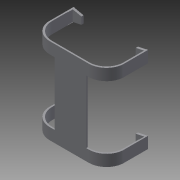
# Autodesk Inventor part: tapa
Saved by Autodesk Inventor 2013 (Build 170138000, 138)
## iProperties
Created: 2013-05-01
Part Number: tapa
Material: Generic
Document SubType Name: Modeling
Designer: otrab
Density: 1 g/cm^3
Author: otrab
Autodesk Inventor part; units mm, degrees
ref_plane "YZ Plane" through (0, 0, 0) normal (1, 0, 0) x (0, 1, 0)
ref_plane "XZ Plane" through (0, 0, 0) normal (0, 1, 0) x (-1, 0, 0)
ref_plane "XY Plane" through (0, 0, 0) normal (0, 0, 1) x (1, 0, 0)
sketch "Sketch1" plane through (0, 0, 0) normal (0, 1, 0) x (-1, 0, 0)
  line L0 (-26, -31) -> (26, -31)
  line L1 (26, -31) -> (26, 31)
  line L2 (26, 31) -> (-26, 31)
  line L3 (-26, 31) -> (-26, -31)
  line L4 (-26, -31) -> (26, 31) construction
  line L5 (26, -31) -> (-26, 31) construction
  point P0 (0, 0)
  dimension "d0" = 52
  dimension "d2" = 62
  constraints: 12 end point, 2 midpoint, 2 parallel, 1 horizontal, 1 perpendicular
  measures "d0" distance of L1.end L2.end
  measures "d2" distance of L2.end L0.start
extrude "Extrusion1" add sketch "Sketch1" along normal blind 1
sketch "Sketch2" plane through (0, 1, 0) normal (0, 1, 0) x (1, 0, 0)
  line L0 (26, 31) -> (-26, 31) projected
  line L1 (-26, 31) -> (-26, -31) projected
  line L2 (-26, -31) -> (26, -31) projected
  line L3 (-26, 31) -> (-25, 31)
  line L4 (-25, 31) -> (-25, -31)
  line L5 (-26, -31) -> (-25, -31)
  line L6 (-26, -31) -> (-26, 31)
  line L7 (0, 46.5401) -> (0, -49.8176) construction
  line L8 (26, 31) -> (26, -31)
  line L9 (26, 31) -> (25, 31)
  line L10 (25, 31) -> (25, -31)
  line L11 (26, -31) -> (25, -31)
  line L12 (26, -31) -> (26, 31)
  point P0 (0, 0)
  dimension "d5" = 1
  constraints: 20 end point, 3 perpendicular, 2 point on line, 2 symmetric about line, 1 parallel
  measures "d5" distance of L0.end L3.end
extrude "Extrusion2" add sketch "Sketch2" along normal blind 28 contours L8 L2 L10 L0 | L4 L2 L1 L0
fillet "Fillet1" radius 12 1 edges at (-25, 1, 0)
mirror "Mirror1" about plane through (0, 0, 0) normal (1, 0, 0) of "Fillet1"
sketch "Sketch3" plane through (-26, 0, -31) normal (-1, 0, 0) x (0, 0, 1)
  line L0 (0, 0) -> (62, 0) projected
  line L1 (62, 29) -> (61, 29) construction
  line L2 (61, 29) -> (61, 27.5)
  line L3 (61, 27.5) -> (53, 27.5)
  line L4 (53, 27.5) -> (53, 29)
  line L5 (61, 29) -> (53, 29)
  line L6 (53, 29) -> (61, 29)
  point P0 (31, 0)
  dimension "d9" = 1
  dimension "d10" = 1.5
  dimension "d11" = 8
  constraints: 12 end point, 1 parallel, 1 perpendicular
  measures "d9" distance of L1.start L1.end
  measures "d10" distance of L1.end L2.end
  measures "d11" distance of L2.end L3.end
extrude "Extrusion3" add sketch "Sketch3" against normal blind 7
mirror "Mirror3" about plane through (0, 0, 0) normal (0, 0, 1) of "Extrusion3"
mirror "Mirror4" about plane through (0, 0, 0) normal (1, 0, 0) of "Extrusion3", "Mirror3"
sketch "Sketch6" plane through (0, 29, 0) normal (0, 1, 0) x (1, 0, 0)
  line L0 (-30.2809, -30.0039) -> (31.8564, -30.0039)
  line L1 (31.8564, -30.0039) -> (31.8564, -41.1164)
  line L2 (31.8564, -41.1164) -> (-30.2809, -41.1164)
  line L3 (-30.2809, -41.1164) -> (-30.2809, -30.0039)
  line L4 (-30.2809, 39.7218) -> (31.1002, 39.7218)
  line L5 (31.1002, 39.7218) -> (31.1002, 29.9909)
  line L6 (31.1002, 29.9909) -> (-30.2809, 29.9909)
  line L7 (-30.2809, 29.9909) -> (-30.2809, 39.7218)
  line L8 (-30.2809, 22.0008) -> (-10.2809, 22.0008)
  line L9 (-10.2809, 22.0008) -> (-10.2809, -21.9612)
  line L10 (-10.2809, -21.9612) -> (-30.2809, -21.9612)
  line L11 (-30.2809, -21.9612) -> (-30.2809, 22.0008)
  line L12 (31.8564, -21.9503) -> (11.8564, -21.9503)
  line L13 (11.8564, -21.9503) -> (11.8564, 22.0008)
  line L14 (11.8564, 22.0008) -> (31.8564, 22.0008)
  line L15 (31.8564, 22.0008) -> (31.8564, -21.9503)
  point P0 (0, 0)
  dimension "d26" = 20
  dimension "d27" = 20
  constraints: 32 end point, 8 parallel, 4 horizontal, 4 perpendicular, 1 collinear
  measures "d26" distance of L9.end L10.end
  measures "d27" distance of L13.end L14.end
extrude "Extrusion6" cut sketch "Sketch6" against normal through all
sketch "Sketch7" plane through (0, 29, 0) normal (0, 1, 0) x (1, 0, 0)
  line L0 (19, 22.0008) -> (19, 30) projected
  line L1 (26, 22.0008) -> (26, 29.9909) projected
  line L2 (19, 30) -> (19, 28.5)
  line L3 (19, 28.5) -> (26, 30)
  line L4 (19, 30) -> (26, 30)
  line L5 (19, 30) -> (19, 22.0008) construction
  line L6 (18.3, 25.9838) -> (30.5903, 25.9838) construction
  line L7 (19, 29.9668) -> (19, 21.9676)
  line L8 (26, 29.9668) -> (26, 21.9767)
  line L9 (19, 21.9676) -> (19, 23.4676)
  line L10 (19, 23.4676) -> (26, 21.9676)
  line L11 (19, 21.9676) -> (26, 21.9676)
  line L12 (19, 21.9676) -> (19, 29.9668) construction
  point P0 (0, 0)
  dimension "d30" = 1.5
  constraints: 22 end point, 6 symmetric about line, 4 point on line, 2 perpendicular, 1 collinear
  measures "d30" distance of L0.end L2.end
extrude "Extrusion7" cut sketch "Sketch7" against normal blind 5
mirror "Mirror6" about plane through (0, 0, 0) normal (1, 0, 0) of "Extrusion7"
mirror "Mirror7" about plane through (0, 0, 0) normal (0, 0, 1) of "Extrusion7", "Mirror6"
sketch "Sketch8" plane through (-26, 0, 30.0039) normal (0, 0, 1) x (1, 0, 0)
  line L0 (0, 0) -> (0, 29) projected
  line L1 (52, 0) -> (0, 0) projected
  line L2 (51, 29) -> (52, 29) projected
  arc A0 (0, 13.6957) -> (12.3777, 0) centre (12.3777, 12.4411) ccw
  line L3 (0, 11.1866) -> (0, 0)
  arc A1 (1, 13) -> (13, 1) centre (13, 13) ccw projected
  line L4 (52, 29) -> (52, 0) projected
  line L5 (26, 0) -> (26, 62.522) construction
  line L6 (52, 0) -> (52, 29)
  line L7 (0, 0) -> (52, 0)
  arc A2 (39.6223, 0) -> (52, 13.6957) centre (39.6223, 12.4411) ccw
  line L8 (52, 11.1866) -> (52, 0)
  arc A3 (39, 1) -> (51, 13) centre (39, 13) ccw
  constraints: 10 end point, 8 point on circle, 7 symmetric about line, 6 point on line, 3 centre point, 1 parallel, 1 perpendicular, 1 tangent, 2 other
extrude "Extrusion8" cut sketch "Sketch8" against normal through all contours L0 A0 L1 | L1 A2 L4
body "Solid1"
